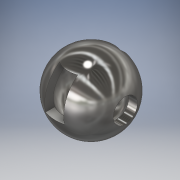
# Autodesk Inventor part: Шар Модель ДЗ
Saved by Autodesk Inventor 2019 (Build 230136000, 136)
## iProperties
Created: 2020-04-11
Part Number: Шар Модель ДЗ
Material: Сталь, высокопрочная, низколегированная
Document SubType Name: Modeling
Designer: Ivan
Mass: 1310.1 g
Surface Area: 388.266 cm^2
Volume: 166.892 cm^3
Density: 7.85 g/cm^3
Appearance: Сталь — полированная
Author: Ivan
Autodesk Inventor part; units mm, degrees
ref_plane "YZ Plane" through (0, 0, 0) normal (1, 0, 0) x (0, 1, 0)
ref_plane "XZ Plane" through (0, 0, 0) normal (0, 1, 0) x (-1, 0, 0)
ref_plane "XY Plane" through (0, 0, 0) normal (0, 0, 1) x (1, 0, 0)
sketch "Эскиз1" plane through (0, 0, 0) normal (0, 0, 1) x (1, 0, 0)
  arc A0 (35, 0) -> (-35, 0) centre (0, 0) ccw
  arc A1 (45, 0) -> (-45, 0) centre (0, 0) ccw
  line L0 (-63, 0) -> (63, 0) projected
  dimension "d0" = 70
  dimension "d1" = 90
  constraints: 4 point on circle, 4 point on line, 2 centre point, 2 coincident
  measures "d0" diameter of A0
  measures "d1" diameter of A1
revolve "Вращение1" add sketch "Эскиз1" angle 360 about axis through (-10, 0, 0) along (1, 0, 0) contours A0 L0 A1
sketch "Эскиз2" plane through (0, 0, 0) normal (0, 0, 1) x (1, 0, 0)
  line L0 (-15, 35) -> (10, 35)
  line L1 (10, 35) -> (10, -10)
  line L2 (10, -10) -> (-15, -10)
  line L3 (-15, -10) -> (-15, 35)
  circle A0 centre (0, 0) radius 35 projected
  dimension "d3" = 25
  dimension "d4" = 10
  dimension "d5" = 45
  dimension "d6" = 10
  constraints: 8 end point, 2 parallel, 1 horizontal, 1 perpendicular
  measures "d3" distance between parallel lines of L1 L3
  measures "d4" distance from line of point (0, 0) L1
  measures "d5" distance between parallel lines of L0 L2
  measures "d6" distance from line of point (0, 0) L2
extrude "Выдавливание1" cut sketch "Эскиз2" along normal through all both and the other way through all contours L0 A0 L3 | L0 L1 A0 | A0 L1 L2 L3 picked at (-5.0617, 4.4951)
sketch "Эскиз3" plane through (0, 0, 0) normal (1, 0, 0) x (0, 1, 0)
  circle A0 centre (0, 0) radius 15
  dimension "d9" = 30
  constraints: 1 centre point, 1 coincident
  measures "d9" diameter of A0
extrude "Выдавливание2" cut sketch "Эскиз3" along normal through all
sketch "Эскиз4" plane through (0, 0, 0) normal (1, 0, 0) x (0, 1, 0)
  point P0 (0, 0)
